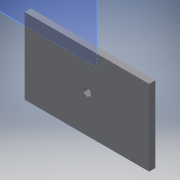
# Autodesk Inventor part: jalador
Saved by Autodesk Inventor 2018.3 (Build 223284000, 284)
## iProperties
Created: 2019-02-25
Part Number: jalador
Material: Generic
Document SubType Name: Modeling
Designer: Mario
Density: 1 g/cm^3
Appearance: Default
Author: Mario
Autodesk Inventor part; units mm, degrees
note: some values were not read from the file. Chosen so that the rebuilt part matches the saved one: direction of "Hole1".
ref_plane "YZ Plane" through (0, 0, 0) normal (1, 0, 0) x (0, 1, 0)
ref_plane "XZ Plane" through (0, 0, 0) normal (0, 1, 0) x (-1, 0, 0)
ref_plane "XY Plane" through (0, 0, 0) normal (0, 0, 1) x (1, 0, 0)
sketch "Sketch1" plane through (0, 0, 0) normal (0, 1, 0) x (-1, 0, 0)
  line L0 (50, 30.5) -> (-50, 30.5)
  line L1 (-50, 30.5) -> (-50, -30.5)
  line L2 (-50, -30.5) -> (50, -30.5)
  line L3 (50, -30.5) -> (50, 30.5)
  line L4 (50, 30.5) -> (-50, -30.5) construction
  line L5 (-50, 30.5) -> (50, -30.5) construction
  point P0 (0, 0)
  dimension "d4" = 61
  dimension "d5" = 100
  constraints: 12 end point, 2 midpoint, 2 parallel, 1 horizontal, 1 perpendicular
  measures "d4" distance of L0.end L1.end
  measures "d5" distance of L0.start L0.end
extrude "Extrusion1" add sketch "Sketch1" along normal blind 5
sketch "Sketch2" plane through (0, 5, 0) normal (0, 1, 0) x (1, 0, 0)
  point P0 (0, 0)
hole "Hole1" at (0, 5, 0) direction (0, -1, 0) diameter 8 end up to surface
body "Solid1"
